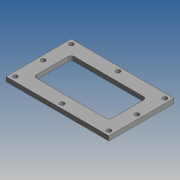
# Autodesk Inventor part: P021_HautEcranProtecLidar
Saved by Autodesk Inventor 2021.3 (Build 253353000, 353)
## iProperties
Created: 2021-11-12
Part Number: P021_HautEcranProtecLidar
Material: Générique
Document SubType Name: Modeling
Designer: gabri
Density: 1 g/cm^3
Appearance: Par défaut
Author: gabri
Autodesk Inventor part; units mm, degrees
ref_plane "YZ Plane" through (0, 0, 0) normal (1, 0, 0) x (0, 1, 0)
ref_plane "XZ Plane" through (0, 0, 0) normal (0, 1, 0) x (-1, 0, 0)
ref_plane "XY Plane" through (0, 0, 0) normal (0, 0, 1) x (1, 0, 0)
sketch "Sketch2" plane through (0, 0, 0) normal (0, 0, 1) x (1, 0, 0)
  line L0 (34, -21.5) -> (-34, -21.5)
  line L1 (-34, -21.5) -> (-34, 21.5)
  line L2 (-34, 21.5) -> (34, 21.5)
  line L3 (34, 21.5) -> (34, -21.5)
  line L4 (34, -21.5) -> (-34, 21.5) construction
  line L5 (-34, -21.5) -> (34, 21.5) construction
  line L6 (23, -12.5) -> (-23, -12.5)
  line L7 (-25, -10.5) -> (-25, 10.5)
  line L8 (-23, 12.5) -> (23, 12.5)
  line L9 (25, 10.5) -> (25, -10.5)
  line L10 (25, -12.5) -> (-25, 12.5) construction
  line L11 (-25, -12.5) -> (25, 12.5) construction
  arc A0 (-23, 12.5) -> (-25, 10.5) centre (-23, 10.5) ccw
  arc A1 (-25, -10.5) -> (-23, -12.5) centre (-23, -10.5) ccw
  arc A2 (23, -12.5) -> (25, -10.5) centre (23, -10.5) ccw
  arc A3 (25, 10.5) -> (23, 12.5) centre (23, 10.5) ccw
  point P0 (0, 0)
  dimension "d0" = 68
  dimension "d1" = 43
  dimension "d4" = 9
  dimension "d5" = 9
  dimension "d6" = 2
  constraints: 24 end point, 8 point on circle, 8 point on line, 8 tangent, 4 centre point, 4 midpoint, 4 parallel, 3 equal radius, 2 horizontal, 2 perpendicular
  measures "d0" distance of L1.end L2.end
  measures "d1" distance of L0.end L1.end
  measures "d4" distance between parallel lines of L2 L8
  measures "d5" distance between parallel lines of L1 L7
  measures "d6" radius of A0
extrude "Extrusion1" add sketch "Sketch2" along normal blind 3
sketch "Sketch3" plane through (0, 0, 3) normal (0, 0, 1) x (1, 0, 0)
  line L0 (-34, -21.5) -> (34, -21.5) construction
  line L1 (34, -21.5) -> (34, 21.5) construction
  line L2 (-34, 21.5) -> (-34, -21.5) construction
  line L3 (34, 21.5) -> (-34, 21.5) construction
  line L4 (-47.6, 0) -> (47.6, 0) construction
  line L5 (0, 30.1) -> (0, -30.1) construction
  line L6 (25, 10.5) -> (25, -10.5) construction
  line L7 (-23, 12.5) -> (23, 12.5) construction
  line L8 (-25, -10.5) -> (-25, 10.5) construction
  line L9 (23, -12.5) -> (-23, -12.5) construction
  point P0 (0, 0)
  point P1 (31, -18.5)
  point P2 (31, 0)
  point P3 (31, 18.5)
  point P4 (0, 18.5)
  point P5 (-31, 18.5)
  point P6 (-31, 0)
  point P7 (-31, -18.5)
  point P8 (0, -18.5)
  dimension "d26" = 6
  dimension "d27" = 6
  dimension "d28" = 6
  dimension "d29" = 6
  dimension "d30" = 6
  dimension "d31" = 6
  dimension "d32" = 6
  dimension "d33" = 6
  dimension "d34" = 6
  dimension "d35" = 6
  dimension "d36" = 6
  dimension "d37" = 6
  constraints: 4 point on line
  measures "d26" distance from line of L6 point (31, 0)
  measures "d27" distance from line of L6 point (31, 18.5)
  measures "d28" distance from line of L7 point (31, 18.5)
  measures "d29" distance from line of L7 point (0, 18.5)
  measures "d30" distance from line of point (-31, 18.5) L7
  measures "d31" distance from line of point (-31, 18.5) L8
  measures "d32" distance from line of L8 point (-31, 0)
  measures "d33" distance from line of L8 point (-31, -18.5)
  measures "d34" distance from line of point (-31, -18.5) L9
  measures "d35" distance from line of L9 point (0, -18.5)
  measures "d36" distance from line of L9 point (31, -18.5)
  measures "d37" distance from line of L6 point (31, -18.5)
hole "Hole1" at (31, -18.5, 3) at (31, 0, 3) at (31, 18.5, 3) at (0, 18.5, 3) at (-31, 18.5, 3) at (-31, 0, 3) at (-31, -18.5, 3) at (0, -18.5, 3) direction (0, 0, -1) diameter 3 depth 8.8 tip angle 118
body "Solid1"
